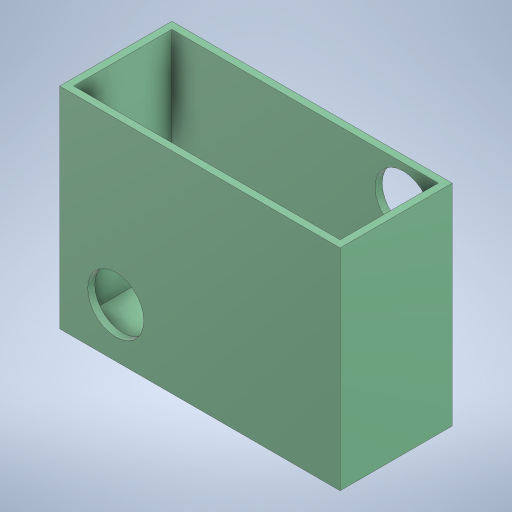
# Autodesk Inventor part: caja de cambios
Saved by Autodesk Inventor 2023 (Build 270158030, 158C)
## iProperties
Created: 2022-05-25
Part Number: caja de cambios
Material: Genérico
Document SubType Name: Modeling
Designer: isaac
Density: 1 g/cm^3
Appearance: Valor por defecto
Author: isaac
Autodesk Inventor part; units mm, degrees
ref_plane "YZ Plane" through (0, 0, 0) normal (1, 0, 0) x (0, 1, 0)
ref_plane "XZ Plane" through (0, 0, 0) normal (0, 1, 0) x (-1, 0, 0)
ref_plane "XY Plane" through (0, 0, 0) normal (0, 0, 1) x (1, 0, 0)
sketch "Boceto1" plane through (0, 0, 0) normal (0, 0, 1) x (1, 0, 0)
  line L0 (-200, 150) -> (200, 150)
  line L1 (200, 150) -> (200, -150)
  line L2 (200, -150) -> (-200, -150)
  line L3 (-200, -150) -> (-200, 150)
  point P0 (0, 0)
  point P1 (0, 150)
  point P2 (-200, 0)
  dimension "d0" = 400
  dimension "d1" = 300
  constraints: 8 end point, 2 midpoint, 2 parallel, 1 horizontal, 1 horizontal alignment, 1 perpendicular, 1 vertical alignment
  measures "d0" distance of L1.end L2.end
  measures "d1" distance of L0.end L1.end
extrude "Extrusión1" add sketch "Boceto1" along normal blind 160
sketch "Boceto2" plane through (-200, 150, 0) normal (0, 1, 0) x (1, 0, 0)
  line L0 (400, 0) -> (0, 0) construction
  line L1 (0, 0) -> (0, -160) construction
  line L2 (400, -160) -> (0, -160) construction
  line L3 (400, 0) -> (400, -160) construction
  line L4 (10, -150) -> (10, -10)
  line L5 (10, -10) -> (390, -10)
  line L6 (390, -10) -> (390, -150)
  line L7 (390, -150) -> (10, -150)
  point P0 (200, 0)
  dimension "d4" = 10
  constraints: 8 end point, 3 other
  measures "d4" distance between parallel lines of L1 L4
extrude "Extrusión2" cut sketch "Boceto2" against normal blind 290
sketch "Boceto3" plane through (0, 0, 160) normal (0, 0, 1) x (1, 0, 0)
  line L0 (-200, -150) -> (200, -150) construction
  line L1 (200, -150) -> (200, 150) construction
  line L2 (200, 150) -> (-200, 150) construction
  line L3 (-200, 150) -> (-200, -150) construction
  circle A0 centre (-120, -80) radius 40
  point P0 (0, 0)
  dimension "d7" = 80
  dimension "d8" = 80
  dimension "d9" = 70
  constraints: 1 centre point
  measures "d7" diameter of A0
  measures "d8" horizontal distance of L0.start A0.centre
  measures "d9" distance from line of L0 A0.centre
extrude "Extrusión3" cut sketch "Boceto3" against normal blind 10
sketch "Boceto4" plane through (0, 0, 0) normal (0, 0, -1) x (-1, 0, 0)
  circle A0 centre (-140, 100) radius 40
  line L0 (200, -150) -> (-200, -150) construction
  line L1 (200, 150) -> (200, -150) construction
  line L2 (-200, 150) -> (200, 150) construction
  line L3 (-200, -150) -> (-200, 150) construction
  point P0 (0, 0)
  dimension "d12" = 80
  dimension "d13" = 50
  dimension "d14" = 60
  constraints: 1 centre point
  measures "d12" diameter of A0
  measures "d13" distance from line of L2 A0.centre
  measures "d14" distance from line of L3 A0.centre
extrude "Extrusión4" cut sketch "Boceto4" against normal blind 10
